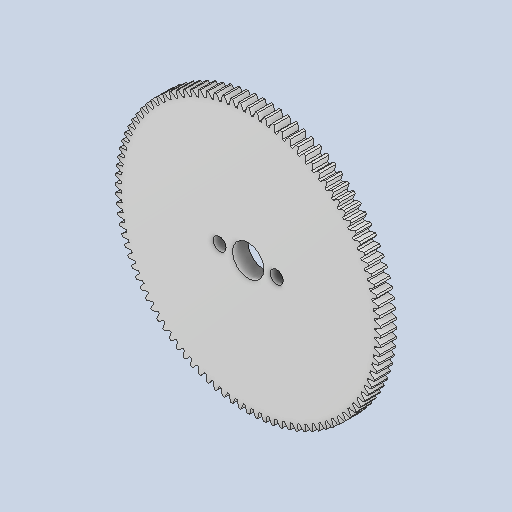
# Autodesk Inventor part: 平歯車1
Saved by Autodesk Inventor 2025.2 (Build 292293000, 293)
## iProperties
CustomPartVersion: 1
Created: 2025-01-13
Part Number: 平歯車1
Material: ABS プラスチック
Document SubType Name: Modeling
Designer: haruy
Categories: <?xml version="1.0" encoding="UTF-16"?> <MemberInstance><Categories><FamilyTemplate><FamilyTemplateParameter ValueType="xs:double" Id="1" ObjectReferenceKey="da_z" ObjectType="kUserParameterObject"/><FamilyTemplateParameter ValueType="xs:double" Id="2" ObjectReferenceKey="da_b" ObjectType="kUserParameterObject"/><FamilyTemplateParameter ValueType="xs:double" Id="3" ObjectReferenceKey="da_beta" ObjectType="kUserParameterObject"/><FamilyTemplateParameter ValueType="xs:double" Id="4" ObjectReferenceKey="da_da" ObjectType="kUserParameterObject"/><FamilyTemplateParameter ValueType="xs:double" Id="5" ObjectReferenceKey="da_aw" ObjectType="kUserParameterObject"/><FamilyTemplateParameter ValueType="xs:string" Id="6" ObjectReferenceKey="EAIAABAAAACIAQAAAAAAAIAAAAAAAAAA" ObjectType="83910656" SubObjectId="SurfaceGeometry"/></FamilyTemplate><ParamToTemplateMap><ParamToTemplate CategoryParameter="//CategoryParameter[@InternalName='046C89C9-8512-4d59-83FE-43B91F4F132A']" TemplateParameter="1"/><ParamToTemplate CategoryParameter="//CategoryParameter[@InternalName='2552DF32-E462-4b46-AEBF-C6C7768E72AC']" TemplateParameter="2"/><ParamToTemplate CategoryParameter="//CategoryParameter[@InternalName='C9EE641D-15FC-4fae-A226-E94C4372FDD7']" TemplateParameter="3"/><ParamToTemplate><ParamToTemplate CategoryParameter="//CategoryParameter[@InternalName='00B6519A-459B-49c7-AD84-2E56D39A5744']" ConstantValue="0.000000"/></ParamToTemplate><ParamToTemplate><ParamToTemplate CategoryParameter="//CategoryParameter[@InternalName='04B31F0E-C7A6-4894-AA32-9629BEFACF47']" ConstantValue="1.000000"/></ParamToTemplate><ParamToTemplate><ParamToTemplate CategoryParameter="//CategoryParameter[@InternalName='43CBEC2E-7847-49e7-A936-2F7889FCB2D9']" ConstantValue="0.250000"/></ParamToTemplate><ParamToTemplate><ParamToTemplate CategoryParameter="//CategoryParameter[@InternalName='B1EFC894-105D-4ebd-86BF-FA20ED196853']" ConstantValue="0.350000"/></ParamToTemplate><ParamToTemplate><ParamToTemplate CategoryParameter="//CategoryParameter[@InternalName='51175063-3D10-4879-93E8-6246FE8B403D']" ConstantValue="2060000000.000000"/></ParamToTemplate><ParamToTemplate><ParamToTemplate CategoryParameter="//CategoryParameter[@InternalName='A3A52E27-4454-46a9-B0BD-C932399B70AF']" ConstantValue="0.300000"/></ParamToTemplate><ParamToTemplate><ParamToTemplate CategoryParameter="//CategoryParameter[@InternalName='91B76062-C214-41d9-B1B9-14D2AB99603D']" ConstantValue="0.100000"/></ParamToTemplate><ParamToTemplate><ParamToTemplate CategoryParameter="//CategoryParameter[@InternalName='374E806E-8B8A-4dda-A9AA-1039D6500AD2']" ConstantValue="10.000000"/></ParamToTemplate><ParamToTemplate><ParamToTemplate CategoryParameter="//CategoryParameter[@InternalName='2D373A89-B862-43d6-8D0B-0CBF12AB9F6C']" ConstantValue="0.349066"/></ParamToTemplate><ParamToTemplate CategoryParameter="//CategoryParameter[@InternalName='37777632-D6A2-4fac-9D53-DB8ACD95C989']" TemplateParameter="4"/><ParamToTemplate CategoryParameter="//CategoryParameter[@InternalName='FD1017F1-B727-4f7e-9707-0F86F1FF9423']" TemplateParameter="5"/><ParamToTemplate><ParamToTemplate CategoryParameter="//CategoryParameter[@InternalName='9E1B4470-B2D3-4ff1-B813-535BB4CDF51A']" ConstantValue="3520000.000000"/></ParamToTemplate><ParamToTemplate><ParamToTemplate CategoryParameter="//CategoryParameter[@InternalName='F8452263-BFF6-458c-9FB1-07C4B99E95CD']" ConstantValue="11400000.000000"/></ParamToTemplate><ParamToTemplate><ParamToTemplate CategoryParameter="//CategoryParameter[@InternalName='3E3BB259-FD49-497f-8171-6EBC954A3479']" ConstantValue="2.000000"/></ParamToTemplate><ParamToTemplate CategoryParameter="//CategoryParameter[@InternalName='27C3BAF2-7550-4e4b-AE2C-0DB134B7D9B7']" TemplateParameter="6"/></ParamToTemplateMap><Category DisplayName="Gear" InternalName="DC85795E-93AB-48d5-8EEE-5A27447B64BD" Mnemonic="Gear"><CategoryParameter DisplayName="z" InternalName="046C89C9-8512-4d59-83FE-43B91F4F132A" Mnemonic="z"/><CategoryParameter DisplayName="b" InternalName="2552DF32-E462-4b46-AEBF-C6C7768E72AC" Mnemonic="b"/><CategoryParameter DisplayName="||b|" InternalName="C9EE641D-15FC-4fae-A226-E94C4372FDD7" Mnemonic="beta"/><CategoryParameter DisplayName="x" InternalName="00B6519A-459B-49c7-AD84-2E56D39A5744" Mnemonic="x"/><CategoryParameter DisplayName="a*" InternalName="04B31F0E-C7A6-4894-AA32-9629BEFACF47" Mnemonic="a"/><CategoryParameter DisplayName="c*" InternalName="43CBEC2E-7847-49e7-A936-2F7889FCB2D9" Mnemonic="c"/><CategoryParameter DisplayName="r|.f|*" InternalName="B1EFC894-105D-4ebd-86BF-FA20ED196853" Mnemonic="rf"/><CategoryParameter DisplayName="E" InternalName="51175063-3D10-4879-93E8-6246FE8B403D" Mnemonic="E"/><CategoryParameter DisplayName="||m|" InternalName="A3A52E27-4454-46a9-B0BD-C932399B70AF" Mnemonic="mi"/><Category DisplayName="SpurGear" InternalName="26C5A22E-A91E-4dfd-A3B3-23CCAFAE1764" Mnemonic="SpurGear"><CategoryParameter DisplayName="m" InternalName="91B76062-C214-41d9-B1B9-14D2AB99603D" Mnemonic="m"/><CategoryParameter DisplayName="P" InternalName="374E806E-8B8A-4dda-A9AA-1039D6500AD2" Mnemonic="PP"/><CategoryParameter DisplayName="||a|" InternalName="2D373A89-B862-43d6-8D0B-0CBF12AB9F6C" Mnemonic="alpha"/><CategoryParameter DisplayName="d|.a|" InternalName="37777632-D6A2-4fac-9D53-DB8ACD95C989" Mnemonic="da"/><CategoryParameter DisplayName="a|.w|" InternalName="FD1017F1-B727-4f7e-9707-0F86F1FF9423" Mnemonic="aw"/><CategoryParameter DisplayName="||s||.Flim|" InternalName="9E1B4470-B2D3-4ff1-B813-535BB4CDF51A" Mnemonic="sFlim"/><CategoryParameter DisplayName="||s||.Hlim|" InternalName="F8452263-BFF6-458c-9FB1-07C4B99E95CD" Mnemonic="sHlim"/><CategoryParameter DisplayName="タイプ" InternalName="3E3BB259-FD49-497f-8171-6EBC954A3479" Mnemonic="type"/><CategoryParameter DisplayName="PitchDiameter" InternalName="27C3BAF2-7550-4e4b-AE2C-0DB134B7D9B7" Mnemonic="IDS_PITCHDIAM"/></Category></Category></Categories></MemberInstance>
Density: 1.06 g/cm^3
Appearance: 滑らか - 白
Author: haruy
Autodesk Inventor part; units mm, degrees
ref_plane "YZ Plane" through (0, 0, 0) normal (1, 0, 0) x (0, 1, 0)
ref_plane "XZ Plane" through (0, 0, 0) normal (0, 1, 0) x (-1, 0, 0)
ref_plane "XY Plane" through (0, 0, 0) normal (0, 0, 1) x (1, 0, 0)
sketch "Sketch1" plane through (0, 0, 0) normal (0, 0, 1) x (1, 0, 0)
  circle A0 centre (0, 0) radius 51
  dimension "d0" = 102
  constraints: 1 centre point
  measures "d0" diameter of A0
extrude "Extrusion1" add sketch "Sketch1" along normal blind 6
ref_plane "Work Plane2" through (0, 0, 3) normal (0, 0, 1) x (1, 0, 0)
sketch "Sketch2" plane through (0, 0, 0) normal (0, 0, -1) x (-1, 0, 0)
  circle A0 centre (0, 0) radius 51 projected
  circle A1 centre (0, 0) radius 50
  dimension "d3" = 100
  constraints: 1 centre point, 1 coincident
  measures "d3" diameter of A1
surface extrude "ピッチ円直径" sketch "Sketch2" against normal through all shown no curves A1
ref_plane "Work Plane8" through (0, 0, 0) normal (0.9995066, 0.0314108, 0) x (0, 0, 1)
ref_plane "Work Plane9" through (0, 0, 0) normal (1, 0, 0) x (0, 1, 0)
spur gear teeth "平歯車" teeth 100 pitch diameter 100 tip diameter 102 root diameter 97.5 face width 6 start plane through (0, 0, 0) normal (0, 0, -1) x (-1, 0, 0)
sketch "スケッチ3" plane through (0, 0, 6) normal (0, 0, 1) x (1, 0, 0)
  circle A0 centre (0, 0) radius 6
  circle A1 centre (0, 0) radius 11
  circle A2 centre (-11, 0) radius 2.5
  circle A3 centre (11, 0) radius 2.5
  dimension "d50" = 22
  dimension "d49" = 12
  dimension "d51" = 5
  dimension "d54" = 360
  constraints: 3 centre point, 2 coincident, 1 horizontal alignment, 7 other
  measures "d49" diameter of A0
  measures "d51" diameter of A2
extrude "押し出し2" cut sketch "スケッチ3" against normal blind 10 contours A0 | A1 A3 | A1 A3 | A2 A1 | A1 A2
sketch "スケッチ4" plane through (0, 0, 6) normal (0, 0, 1) x (1, 0, 0)
  circle A0 centre (11, 0) radius 2.5 projected
  circle A1 centre (-11, 0) radius 2.5 projected
  circle A2 centre (0, 0) radius 6 projected
  arc A3 (-3.602, 50.8726) -> (-4.2065, 48.5682) centre (9.678, 46.1577) ccw projected
  arc A4 (-4.2065, 48.5682) -> (-4.9688, 48.4961) centre (0, 0) ccw projected
  arc A5 (-4.9688, 48.4961) -> (-5.9944, 50.6465) centre (-18.1557, 43.5266) ccw projected
  arc A6 (-5.9944, 50.6465) -> (-6.7892, 50.5461) centre (0, 0) ccw projected
  arc A7 (-6.7892, 50.5461) -> (-7.2478, 48.2082) centre (6.7606, 46.6743) ccw projected
  arc A8 (-7.2478, 48.2082) -> (-8.0041, 48.0884) centre (0, 0) ccw projected
  arc A9 (-8.0041, 48.0884) -> (-9.1627, 50.1702) centre (-20.8529, 42.3007) ccw projected
  arc A10 (-9.1627, 50.1702) -> (-9.9496, 50.02) centre (0, 0) ccw projected
  arc A11 (-9.9496, 50.02) -> (-10.2605, 47.658) centre (3.8166, 47.0067) ccw projected
  arc A12 (-10.2605, 47.658) -> (-11.0078, 47.491) centre (0, 0) ccw projected
  arc A13 (-11.0078, 47.491) -> (-12.2948, 49.4958) centre (-23.4678, 40.9079) ccw projected
  arc A14 (-12.2948, 49.4958) -> (-13.0708, 49.2966) centre (0, 0) ccw projected
  arc A15 (-13.0708, 49.2966) -> (-13.2327, 46.9197) centre (0.8575, 47.1536) ccw projected
  arc A16 (-13.2327, 46.9197) -> (-13.9681, 46.7061) centre (0, 0) ccw projected
  arc A17 (-13.9681, 46.7061) -> (-15.3784, 48.6262) centre (-25.9901, 39.3536) ccw projected
  arc A18 (-15.3784, 48.6262) -> (-16.1403, 48.3786) centre (0, 0) ccw projected
  arc A19 (-16.1403, 48.3786) -> (-16.1527, 45.9962) centre (-2.105, 47.1143) ccw projected
  arc A20 (-16.1527, 45.9962) -> (-16.8732, 45.7368) centre (0, 0) ccw projected
  arc A21 (-16.8732, 45.7368) -> (-18.4014, 47.5646) centre (-28.4099, 37.644) ccw projected
  arc A22 (-18.4014, 47.5646) -> (-19.1462, 47.2697) centre (0, 0) ccw projected
  arc A23 (-19.1462, 47.2697) -> (-19.009, 44.8912) centre (-5.0592, 46.8892) ccw projected
  arc A24 (-19.009, 44.8912) -> (-19.7118, 44.5871) centre (0, 0) ccw projected
  arc A25 (-19.7118, 44.5871) -> (-21.3516, 46.3153) centre (-30.7175, 35.7859) ccw projected
  arc A26 (-21.3516, 46.3153) -> (-22.0765, 45.9742) centre (0, 0) ccw projected
  arc A27 (-22.0765, 45.9742) -> (-21.7902, 43.6091) centre (-7.9934, 46.479) ccw projected
  arc A28 (-21.7902, 43.6091) -> (-22.4725, 43.2614) centre (0, 0) ccw projected
  arc A29 (-22.4725, 43.2614) -> (-24.2177, 44.8832) centre (-32.9039, 33.7865) ccw projected
  arc A30 (-24.2177, 44.8832) -> (-24.9197, 44.4973) centre (0, 0) ccw projected
  arc A31 (-24.9197, 44.4973) -> (-24.4854, 42.1548) centre (-10.8961, 45.8854) ccw projected
  arc A32 (-24.4854, 42.1548) -> (-25.1446, 41.765) centre (0, 0) ccw projected
  arc A33 (-25.1446, 41.765) -> (-26.9881, 43.274) centre (-34.9605, 31.6537) ccw projected
  arc A34 (-26.9881, 43.274) -> (-27.6645, 42.8448) centre (0, 0) ccw projected
  arc A35 (-27.6645, 42.8448) -> (-27.084, 40.5341) centre (-13.7557, 45.1107) ccw projected
  arc A36 (-27.084, 40.5341) -> (-27.7174, 40.1037) centre (0, 0) ccw projected
  arc A37 (-27.7174, 40.1037) -> (-29.6521, 41.494) centre (-36.879, 29.3961) ccw projected
  arc A38 (-29.6521, 41.494) -> (-30.3002, 41.0232) centre (0, 0) ccw projected
  arc A39 (-30.3002, 41.0232) -> (-29.5758, 38.7535) centre (-16.5611, 44.1579) ccw projected
  arc A40 (-29.5758, 38.7535) -> (-30.1808, 38.2842) centre (0, 0) ccw projected
  arc A41 (-30.1808, 38.2842) -> (-32.199, 39.5503) centre (-38.652, 27.0224) ccw projected
  arc A42 (-32.199, 39.5503) -> (-32.8162, 39.0396) centre (0, 0) ccw projected
  arc A43 (-32.8162, 39.0396) -> (-31.9508, 36.82) centre (-19.3011, 43.0309) ccw projected
  arc A44 (-31.9508, 36.82) -> (-32.5252, 36.3136) centre (0, 0) ccw projected
  arc A45 (-32.5252, 36.3136) -> (-34.6188, 37.4504) centre (-40.2725, 24.5421) ccw projected
  arc A46 (-34.6188, 37.4504) -> (-35.2028, 36.9021) centre (0, 0) ccw projected
  arc A47 (-35.2028, 36.9021) -> (-34.1997, 34.7411) centre (-21.965, 41.7341) ccw projected
  arc A48 (-34.1997, 34.7411) -> (-34.7411, 34.1997) centre (0, 0) ccw projected
  arc A49 (-34.7411, 34.1997) -> (-36.9021, 35.2028) centre (-41.7341, 21.965) ccw projected
  arc A50 (-36.9021, 35.2028) -> (-37.4504, 34.6188) centre (0, 0) ccw projected
  arc A51 (-37.4504, 34.6188) -> (-36.3136, 32.5252) centre (-24.5421, 40.2725) ccw projected
  arc A52 (-36.3136, 32.5252) -> (-36.82, 31.9508) centre (0, 0) ccw projected
  arc A53 (-36.82, 31.9508) -> (-39.0396, 32.8162) centre (-43.0309, 19.3011) ccw projected
  arc A54 (-39.0396, 32.8162) -> (-39.5503, 32.199) centre (0, 0) ccw projected
  arc A55 (-39.5503, 32.199) -> (-38.2842, 30.1808) centre (-27.0224, 38.652) ccw projected
  arc A56 (-38.2842, 30.1808) -> (-38.7535, 29.5758) centre (0, 0) ccw projected
  arc A57 (-38.7535, 29.5758) -> (-41.0232, 30.3002) centre (-44.1579, 16.5611) ccw projected
  arc A58 (-41.0232, 30.3002) -> (-41.494, 29.6521) centre (0, 0) ccw projected
  arc A59 (-41.494, 29.6521) -> (-40.1037, 27.7174) centre (-29.3961, 36.879) ccw projected
  arc A60 (-40.1037, 27.7174) -> (-40.5341, 27.084) centre (0, 0) ccw projected
  arc A61 (-40.5341, 27.084) -> (-42.8448, 27.6645) centre (-45.1107, 13.7557) ccw projected
  arc A62 (-42.8448, 27.6645) -> (-43.274, 26.9881) centre (0, 0) ccw projected
  arc A63 (-43.274, 26.9881) -> (-41.765, 25.1446) centre (-31.6537, 34.9605) ccw projected
  arc A64 (-41.765, 25.1446) -> (-42.1548, 24.4854) centre (0, 0) ccw projected
  arc A65 (-42.1548, 24.4854) -> (-44.4973, 24.9197) centre (-45.8854, 10.8961) ccw projected
  arc A66 (-44.4973, 24.9197) -> (-44.8832, 24.2177) centre (0, 0) ccw projected
  arc A67 (-44.8832, 24.2177) -> (-43.2614, 22.4725) centre (-33.7865, 32.9039) ccw projected
  arc A68 (-43.2614, 22.4725) -> (-43.6091, 21.7902) centre (0, 0) ccw projected
  arc A69 (-43.6091, 21.7902) -> (-45.9742, 22.0765) centre (-46.479, 7.9934) ccw projected
  arc A70 (-45.9742, 22.0765) -> (-46.3153, 21.3516) centre (0, 0) ccw projected
  arc A71 (-46.3153, 21.3516) -> (-44.5871, 19.7118) centre (-35.7859, 30.7175) ccw projected
  arc A72 (-44.5871, 19.7118) -> (-44.8912, 19.009) centre (0, 0) ccw projected
  arc A73 (-44.8912, 19.009) -> (-47.2697, 19.1462) centre (-46.8892, 5.0592) ccw projected
  arc A74 (-47.2697, 19.1462) -> (-47.5646, 18.4014) centre (0, 0) ccw projected
  arc A75 (-47.5646, 18.4014) -> (-45.7368, 16.8732) centre (-37.644, 28.4099) ccw projected
  arc A76 (-45.7368, 16.8732) -> (-45.9962, 16.1527) centre (0, 0) ccw projected
  arc A77 (-45.9962, 16.1527) -> (-48.3786, 16.1403) centre (-47.1143, 2.105) ccw projected
  arc A78 (-48.3786, 16.1403) -> (-48.6262, 15.3784) centre (0, 0) ccw projected
  arc A79 (-48.6262, 15.3784) -> (-46.7061, 13.9681) centre (-39.3536, 25.9901) ccw projected
  arc A80 (-46.7061, 13.9681) -> (-46.9197, 13.2327) centre (0, 0) ccw projected
  arc A81 (-46.9197, 13.2327) -> (-49.2966, 13.0708) centre (-47.1536, -0.8575) ccw projected
  arc A82 (-49.2966, 13.0708) -> (-49.4958, 12.2948) centre (0, 0) ccw projected
  arc A83 (-49.4958, 12.2948) -> (-47.491, 11.0078) centre (-40.9079, 23.4678) ccw projected
  arc A84 (-47.491, 11.0078) -> (-47.658, 10.2605) centre (0, 0) ccw projected
  arc A85 (-47.658, 10.2605) -> (-50.02, 9.9496) centre (-47.0067, -3.8166) ccw projected
  arc A86 (-50.02, 9.9496) -> (-50.1702, 9.1627) centre (0, 0) ccw projected
  arc A87 (-50.1702, 9.1627) -> (-48.0884, 8.0041) centre (-42.3007, 20.8529) ccw projected
  arc A88 (-48.0884, 8.0041) -> (-48.2082, 7.2478) centre (0, 0) ccw projected
  arc A89 (-48.2082, 7.2478) -> (-50.5461, 6.7892) centre (-46.6743, -6.7606) ccw projected
  arc A90 (-50.5461, 6.7892) -> (-50.6465, 5.9944) centre (0, 0) ccw projected
  arc A91 (-50.6465, 5.9944) -> (-48.4961, 4.9688) centre (-43.5266, 18.1557) ccw projected
  arc A92 (-48.4961, 4.9688) -> (-48.5682, 4.2065) centre (0, 0) ccw projected
  arc A93 (-48.5682, 4.2065) -> (-50.8726, 3.602) centre (-46.1577, -9.678) ccw projected
  arc A94 (-50.8726, 3.602) -> (-50.9229, 2.8025) centre (0, 0) ccw projected
  arc A95 (-50.9229, 2.8025) -> (-48.7124, 1.9139) centre (-44.5807, 15.3868) ccw projected
  arc A96 (-48.7124, 1.9139) -> (-48.7365, 1.1485) centre (0, 0) ccw projected
  arc A97 (-48.7365, 1.1485) -> (-50.9984, 0.4005) centre (-45.4589, -12.5572) ccw projected
  arc A98 (-50.9984, 0.4005) -> (-50.9984, -0.4005) centre (0, 0) ccw projected
  arc A99 (-50.9984, -0.4005) -> (-48.7365, -1.1485) centre (-45.4589, 12.5572) ccw projected
  arc A100 (-48.7365, -1.1485) -> (-48.7124, -1.9139) centre (0, 0) ccw projected
  arc A101 (-48.7124, -1.9139) -> (-50.9229, -2.8025) centre (-44.5807, -15.3868) ccw projected
  arc A102 (-50.9229, -2.8025) -> (-50.8726, -3.602) centre (0, 0) ccw projected
  arc A103 (-50.8726, -3.602) -> (-48.5682, -4.2065) centre (-46.1577, 9.678) ccw projected
  arc A104 (-48.5682, -4.2065) -> (-48.4961, -4.9688) centre (0, 0) ccw projected
  arc A105 (-48.4961, -4.9688) -> (-50.6465, -5.9944) centre (-43.5266, -18.1557) ccw projected
  arc A106 (-50.6465, -5.9944) -> (-50.5461, -6.7892) centre (0, 0) ccw projected
  arc A107 (-50.5461, -6.7892) -> (-48.2082, -7.2478) centre (-46.6743, 6.7606) ccw projected
  arc A108 (-48.2082, -7.2478) -> (-48.0884, -8.0041) centre (0, 0) ccw projected
  arc A109 (-48.0884, -8.0041) -> (-50.1702, -9.1627) centre (-42.3007, -20.8529) ccw projected
  arc A110 (-50.1702, -9.1627) -> (-50.02, -9.9496) centre (0, 0) ccw projected
  arc A111 (-50.02, -9.9496) -> (-47.658, -10.2605) centre (-47.0067, 3.8166) ccw projected
  arc A112 (-47.658, -10.2605) -> (-47.491, -11.0078) centre (0, 0) ccw projected
  arc A113 (-47.491, -11.0078) -> (-49.4958, -12.2948) centre (-40.9079, -23.4678) ccw projected
  arc A114 (-49.4958, -12.2948) -> (-49.2966, -13.0708) centre (0, 0) ccw projected
  arc A115 (-49.2966, -13.0708) -> (-46.9197, -13.2327) centre (-47.1536, 0.8575) ccw projected
  arc A116 (-46.9197, -13.2327) -> (-46.7061, -13.9681) centre (0, 0) ccw projected
  arc A117 (-46.7061, -13.9681) -> (-48.6262, -15.3784) centre (-39.3536, -25.9901) ccw projected
  arc A118 (-48.6262, -15.3784) -> (-48.3786, -16.1403) centre (0, 0) ccw projected
  arc A119 (-48.3786, -16.1403) -> (-45.9962, -16.1527) centre (-47.1143, -2.105) ccw projected
  arc A120 (-45.9962, -16.1527) -> (-45.7368, -16.8732) centre (0, 0) ccw projected
  arc A121 (-45.7368, -16.8732) -> (-47.5646, -18.4014) centre (-37.644, -28.4099) ccw projected
  arc A122 (-47.5646, -18.4014) -> (-47.2697, -19.1462) centre (0, 0) ccw projected
  arc A123 (-47.2697, -19.1462) -> (-44.8912, -19.009) centre (-46.8892, -5.0592) ccw projected
  arc A124 (-44.8912, -19.009) -> (-44.5871, -19.7118) centre (0, 0) ccw projected
  arc A125 (-44.5871, -19.7118) -> (-46.3153, -21.3516) centre (-35.7859, -30.7175) ccw projected
  arc A126 (-46.3153, -21.3516) -> (-45.9742, -22.0765) centre (0, 0) ccw projected
  arc A127 (-45.9742, -22.0765) -> (-43.6091, -21.7902) centre (-46.479, -7.9934) ccw projected
  arc A128 (-43.6091, -21.7902) -> (-43.2614, -22.4725) centre (0, 0) ccw projected
  arc A129 (-43.2614, -22.4725) -> (-44.8832, -24.2177) centre (-33.7865, -32.9039) ccw projected
  arc A130 (-44.8832, -24.2177) -> (-44.4973, -24.9197) centre (0, 0) ccw projected
  arc A131 (-44.4973, -24.9197) -> (-42.1548, -24.4854) centre (-45.8854, -10.8961) ccw projected
  arc A132 (-42.1548, -24.4854) -> (-41.765, -25.1446) centre (0, 0) ccw projected
  arc A133 (-41.765, -25.1446) -> (-43.274, -26.9881) centre (-31.6537, -34.9605) ccw projected
  arc A134 (-43.274, -26.9881) -> (-42.8448, -27.6645) centre (0, 0) ccw projected
  arc A135 (-42.8448, -27.6645) -> (-40.5341, -27.084) centre (-45.1107, -13.7557) ccw projected
  arc A136 (-40.5341, -27.084) -> (-40.1037, -27.7174) centre (0, 0) ccw projected
  arc A137 (-40.1037, -27.7174) -> (-41.494, -29.6521) centre (-29.3961, -36.879) ccw projected
  arc A138 (-41.494, -29.6521) -> (-41.0232, -30.3002) centre (0, 0) ccw projected
  arc A139 (-41.0232, -30.3002) -> (-38.7535, -29.5758) centre (-44.1579, -16.5611) ccw projected
  arc A140 (-38.7535, -29.5758) -> (-38.2842, -30.1808) centre (0, 0) ccw projected
  arc A141 (-38.2842, -30.1808) -> (-39.5503, -32.199) centre (-27.0224, -38.652) ccw projected
  arc A142 (-39.5503, -32.199) -> (-39.0396, -32.8162) centre (0, 0) ccw projected
  arc A143 (-39.0396, -32.8162) -> (-36.82, -31.9508) centre (-43.0309, -19.3011) ccw projected
  arc A144 (-36.82, -31.9508) -> (-36.3136, -32.5252) centre (0, 0) ccw projected
  arc A145 (-36.3136, -32.5252) -> (-37.4504, -34.6188) centre (-24.5421, -40.2725) ccw projected
  arc A146 (-37.4504, -34.6188) -> (-36.9021, -35.2028) centre (0, 0) ccw projected
  arc A147 (-36.9021, -35.2028) -> (-34.7411, -34.1997) centre (-41.7341, -21.965) ccw projected
  arc A148 (-34.7411, -34.1997) -> (-34.1997, -34.7411) centre (0, 0) ccw projected
  arc A149 (-34.1997, -34.7411) -> (-35.2028, -36.9021) centre (-21.965, -41.7341) ccw projected
  arc A150 (-35.2028, -36.9021) -> (-34.6188, -37.4504) centre (0, 0) ccw projected
  arc A151 (-34.6188, -37.4504) -> (-32.5252, -36.3136) centre (-40.2725, -24.5421) ccw projected
  arc A152 (-32.5252, -36.3136) -> (-31.9508, -36.82) centre (0, 0) ccw projected
  arc A153 (-31.9508, -36.82) -> (-32.8162, -39.0396) centre (-19.3011, -43.0309) ccw projected
  arc A154 (-32.8162, -39.0396) -> (-32.199, -39.5503) centre (0, 0) ccw projected
  arc A155 (-32.199, -39.5503) -> (-30.1808, -38.2842) centre (-38.652, -27.0224) ccw projected
  arc A156 (-30.1808, -38.2842) -> (-29.5758, -38.7535) centre (0, 0) ccw projected
  arc A157 (-29.5758, -38.7535) -> (-30.3002, -41.0232) centre (-16.5611, -44.1579) ccw projected
  arc A158 (-30.3002, -41.0232) -> (-29.6521, -41.494) centre (0, 0) ccw projected
  arc A159 (-29.6521, -41.494) -> (-27.7174, -40.1037) centre (-36.879, -29.3961) ccw projected
  arc A160 (-27.7174, -40.1037) -> (-27.084, -40.5341) centre (0, 0) ccw projected
  arc A161 (-27.084, -40.5341) -> (-27.6645, -42.8448) centre (-13.7557, -45.1107) ccw projected
  arc A162 (-27.6645, -42.8448) -> (-26.9881, -43.274) centre (0, 0) ccw projected
  arc A163 (-26.9881, -43.274) -> (-25.1446, -41.765) centre (-34.9605, -31.6537) ccw projected
  arc A164 (-25.1446, -41.765) -> (-24.4854, -42.1548) centre (0, 0) ccw projected
  arc A165 (-24.4854, -42.1548) -> (-24.9197, -44.4973) centre (-10.8961, -45.8854) ccw projected
  arc A166 (-24.9197, -44.4973) -> (-24.2177, -44.8832) centre (0, 0) ccw projected
  arc A167 (-24.2177, -44.8832) -> (-22.4725, -43.2614) centre (-32.9039, -33.7865) ccw projected
  arc A168 (-22.4725, -43.2614) -> (-21.7902, -43.6091) centre (0, 0) ccw projected
  arc A169 (-21.7902, -43.6091) -> (-22.0765, -45.9742) centre (-7.9934, -46.479) ccw projected
  arc A170 (-22.0765, -45.9742) -> (-21.3516, -46.3153) centre (0, 0) ccw projected
  arc A171 (-21.3516, -46.3153) -> (-19.7118, -44.5871) centre (-30.7175, -35.7859) ccw projected
  arc A172 (-19.7118, -44.5871) -> (-19.009, -44.8912) centre (0, 0) ccw projected
  arc A173 (-19.009, -44.8912) -> (-19.1462, -47.2697) centre (-5.0592, -46.8892) ccw projected
  arc A174 (-19.1462, -47.2697) -> (-18.4014, -47.5646) centre (0, 0) ccw projected
  arc A175 (-18.4014, -47.5646) -> (-16.8732, -45.7368) centre (-28.4099, -37.644) ccw projected
  arc A176 (-16.8732, -45.7368) -> (-16.1527, -45.9962) centre (0, 0) ccw projected
  arc A177 (-16.1527, -45.9962) -> (-16.1403, -48.3786) centre (-2.105, -47.1143) ccw projected
  arc A178 (-16.1403, -48.3786) -> (-15.3784, -48.6262) centre (0, 0) ccw projected
  arc A179 (-15.3784, -48.6262) -> (-13.9681, -46.7061) centre (-25.9901, -39.3536) ccw projected
  arc A180 (-13.9681, -46.7061) -> (-13.2327, -46.9197) centre (0, 0) ccw projected
  arc A181 (-13.2327, -46.9197) -> (-13.0708, -49.2966) centre (0.8575, -47.1536) ccw projected
  arc A182 (-13.0708, -49.2966) -> (-12.2948, -49.4958) centre (0, 0) ccw projected
  arc A183 (-12.2948, -49.4958) -> (-11.0078, -47.491) centre (-23.4678, -40.9079) ccw projected
  arc A184 (-11.0078, -47.491) -> (-10.2605, -47.658) centre (0, 0) ccw projected
  arc A185 (-10.2605, -47.658) -> (-9.9496, -50.02) centre (3.8166, -47.0067) ccw projected
  arc A186 (-9.9496, -50.02) -> (-9.1627, -50.1702) centre (0, 0) ccw projected
  arc A187 (-9.1627, -50.1702) -> (-8.0041, -48.0884) centre (-20.8529, -42.3007) ccw projected
  arc A188 (-8.0041, -48.0884) -> (-7.2478, -48.2082) centre (0, 0) ccw projected
  arc A189 (-7.2478, -48.2082) -> (-6.7892, -50.5461) centre (6.7606, -46.6743) ccw projected
  arc A190 (-6.7892, -50.5461) -> (-5.9944, -50.6465) centre (0, 0) ccw projected
  arc A191 (-5.9944, -50.6465) -> (-4.9688, -48.4961) centre (-18.1557, -43.5266) ccw projected
  arc A192 (-4.9688, -48.4961) -> (-4.2065, -48.5682) centre (0, 0) ccw projected
  arc A193 (-4.2065, -48.5682) -> (-3.602, -50.8726) centre (9.678, -46.1577) ccw projected
  arc A194 (-3.602, -50.8726) -> (-2.8025, -50.9229) centre (0, 0) ccw projected
  arc A195 (-2.8025, -50.9229) -> (-1.9139, -48.7124) centre (-15.3868, -44.5807) ccw projected
  arc A196 (-1.9139, -48.7124) -> (-1.1485, -48.7365) centre (0, 0) ccw projected
  arc A197 (-1.1485, -48.7365) -> (-0.4005, -50.9984) centre (12.5572, -45.4589) ccw projected
  arc A198 (-0.4005, -50.9984) -> (0.4005, -50.9984) centre (0, 0) ccw projected
  arc A199 (0.4005, -50.9984) -> (1.1485, -48.7365) centre (-12.5572, -45.4589) ccw projected
  arc A200 (1.1485, -48.7365) -> (1.9139, -48.7124) centre (0, 0) ccw projected
  arc A201 (1.9139, -48.7124) -> (2.8025, -50.9229) centre (15.3868, -44.5807) ccw projected
  arc A202 (2.8025, -50.9229) -> (3.602, -50.8726) centre (0, 0) ccw projected
  arc A203 (3.602, -50.8726) -> (4.2065, -48.5682) centre (-9.678, -46.1577) ccw projected
  arc A204 (4.2065, -48.5682) -> (4.9688, -48.4961) centre (0, 0) ccw projected
  arc A205 (4.9688, -48.4961) -> (5.9944, -50.6465) centre (18.1557, -43.5266) ccw projected
  arc A206 (5.9944, -50.6465) -> (6.7892, -50.5461) centre (0, 0) ccw projected
  arc A207 (6.7892, -50.5461) -> (7.2478, -48.2082) centre (-6.7606, -46.6743) ccw projected
  arc A208 (7.2478, -48.2082) -> (8.0041, -48.0884) centre (0, 0) ccw projected
  arc A209 (8.0041, -48.0884) -> (9.1627, -50.1702) centre (20.8529, -42.3007) ccw projected
  arc A210 (9.1627, -50.1702) -> (9.9496, -50.02) centre (0, 0) ccw projected
  arc A211 (9.9496, -50.02) -> (10.2605, -47.658) centre (-3.8166, -47.0067) ccw projected
  arc A212 (10.2605, -47.658) -> (11.0078, -47.491) centre (0, 0) ccw projected
  arc A213 (11.0078, -47.491) -> (12.2948, -49.4958) centre (23.4678, -40.9079) ccw projected
  arc A214 (12.2948, -49.4958) -> (13.0708, -49.2966) centre (0, 0) ccw projected
  arc A215 (13.0708, -49.2966) -> (13.2327, -46.9197) centre (-0.8575, -47.1536) ccw projected
  arc A216 (13.2327, -46.9197) -> (13.9681, -46.7061) centre (0, 0) ccw projected
  arc A217 (13.9681, -46.7061) -> (15.3784, -48.6262) centre (25.9901, -39.3536) ccw projected
  arc A218 (15.3784, -48.6262) -> (16.1403, -48.3786) centre (0, 0) ccw projected
  arc A219 (16.1403, -48.3786) -> (16.1527, -45.9962) centre (2.105, -47.1143) ccw projected
  arc A220 (16.1527, -45.9962) -> (16.8732, -45.7368) centre (0, 0) ccw projected
  arc A221 (16.8732, -45.7368) -> (18.4014, -47.5646) centre (28.4099, -37.644) ccw projected
  arc A222 (18.4014, -47.5646) -> (19.1462, -47.2697) centre (0, 0) ccw projected
  arc A223 (19.1462, -47.2697) -> (19.009, -44.8912) centre (5.0592, -46.8892) ccw projected
  arc A224 (19.009, -44.8912) -> (19.7118, -44.5871) centre (0, 0) ccw projected
  arc A225 (19.7118, -44.5871) -> (21.3516, -46.3153) centre (30.7175, -35.7859) ccw projected
  arc A226 (21.3516, -46.3153) -> (22.0765, -45.9742) centre (0, 0) ccw projected
  arc A227 (22.0765, -45.9742) -> (21.7902, -43.6091) centre (7.9934, -46.479) ccw projected
  arc A228 (21.7902, -43.6091) -> (22.4725, -43.2614) centre (0, 0) ccw projected
  arc A229 (22.4725, -43.2614) -> (24.2177, -44.8832) centre (32.9039, -33.7865) ccw projected
  arc A230 (24.2177, -44.8832) -> (24.9197, -44.4973) centre (0, 0) ccw projected
  arc A231 (24.9197, -44.4973) -> (24.4854, -42.1548) centre (10.8961, -45.8854) ccw projected
  arc A232 (24.4854, -42.1548) -> (25.1446, -41.765) centre (0, 0) ccw projected
  arc A233 (25.1446, -41.765) -> (26.9881, -43.274) centre (34.9605, -31.6537) ccw projected
  arc A234 (26.9881, -43.274) -> (27.6645, -42.8448) centre (0, 0) ccw projected
  arc A235 (27.6645, -42.8448) -> (27.084, -40.5341) centre (13.7557, -45.1107) ccw projected
  arc A236 (27.084, -40.5341) -> (27.7174, -40.1037) centre (0, 0) ccw projected
  arc A237 (27.7174, -40.1037) -> (29.6521, -41.494) centre (36.879, -29.3961) ccw projected
  arc A238 (29.6521, -41.494) -> (30.3002, -41.0232) centre (0, 0) ccw projected
  arc A239 (30.3002, -41.0232) -> (29.5758, -38.7535) centre (16.5611, -44.1579) ccw projected
  arc A240 (29.5758, -38.7535) -> (30.1808, -38.2842) centre (0, 0) ccw projected
  arc A241 (30.1808, -38.2842) -> (32.199, -39.5503) centre (38.652, -27.0224) ccw projected
  arc A242 (32.199, -39.5503) -> (32.8162, -39.0396) centre (0, 0) ccw projected
  arc A243 (32.8162, -39.0396) -> (31.9508, -36.82) centre (19.3011, -43.0309) ccw projected
  arc A244 (31.9508, -36.82) -> (32.5252, -36.3136) centre (0, 0) ccw projected
  arc A245 (32.5252, -36.3136) -> (34.6188, -37.4504) centre (40.2725, -24.5421) ccw projected
  arc A246 (34.6188, -37.4504) -> (35.2028, -36.9021) centre (0, 0) ccw projected
  arc A247 (35.2028, -36.9021) -> (34.1997, -34.7411) centre (21.965, -41.7341) ccw projected
  arc A248 (34.1997, -34.7411) -> (34.7411, -34.1997) centre (0, 0) ccw projected
  arc A249 (34.7411, -34.1997) -> (36.9021, -35.2028) centre (41.7341, -21.965) ccw projected
  arc A250 (36.9021, -35.2028) -> (37.4504, -34.6188) centre (0, 0) ccw projected
  arc A251 (37.4504, -34.6188) -> (36.3136, -32.5252) centre (24.5421, -40.2725) ccw projected
  arc A252 (36.3136, -32.5252) -> (36.82, -31.9508) centre (0, 0) ccw projected
  arc A253 (36.82, -31.9508) -> (39.0396, -32.8162) centre (43.0309, -19.3011) ccw projected
  arc A254 (39.0396, -32.8162) -> (39.5503, -32.199) centre (0, 0) ccw projected
  arc A255 (39.5503, -32.199) -> (38.2842, -30.1808) centre (27.0224, -38.652) ccw projected
  arc A256 (38.2842, -30.1808) -> (38.7535, -29.5758) centre (0, 0) ccw projected
  arc A257 (38.7535, -29.5758) -> (41.0232, -30.3002) centre (44.1579, -16.5611) ccw projected
  arc A258 (41.0232, -30.3002) -> (41.494, -29.6521) centre (0, 0) ccw projected
  arc A259 (41.494, -29.6521) -> (40.1037, -27.7174) centre (29.3961, -36.879) ccw projected
  arc A260 (40.1037, -27.7174) -> (40.5341, -27.084) centre (0, 0) ccw projected
  arc A261 (40.5341, -27.084) -> (42.8448, -27.6645) centre (45.1107, -13.7557) ccw projected
  arc A262 (42.8448, -27.6645) -> (43.274, -26.9881) centre (0, 0) ccw projected
  arc A263 (43.274, -26.9881) -> (41.765, -25.1446) centre (31.6537, -34.9605) ccw projected
  arc A264 (41.765, -25.1446) -> (42.1548, -24.4854) centre (0, 0) ccw projected
  arc A265 (42.1548, -24.4854) -> (44.4973, -24.9197) centre (45.8854, -10.8961) ccw projected
  arc A266 (44.4973, -24.9197) -> (44.8832, -24.2177) centre (0, 0) ccw projected
  arc A267 (44.8832, -24.2177) -> (43.2614, -22.4725) centre (33.7865, -32.9039) ccw projected
  arc A268 (43.2614, -22.4725) -> (43.6091, -21.7902) centre (0, 0) ccw projected
  arc A269 (43.6091, -21.7902) -> (45.9742, -22.0765) centre (46.479, -7.9934) ccw projected
  arc A270 (45.9742, -22.0765) -> (46.3153, -21.3516) centre (0, 0) ccw projected
  arc A271 (46.3153, -21.3516) -> (44.5871, -19.7118) centre (35.7859, -30.7175) ccw projected
  arc A272 (44.5871, -19.7118) -> (44.8912, -19.009) centre (0, 0) ccw projected
  arc A273 (44.8912, -19.009) -> (47.2697, -19.1462) centre (46.8892, -5.0592) ccw projected
  arc A274 (47.2697, -19.1462) -> (47.5646, -18.4014) centre (0, 0) ccw projected
  arc A275 (47.5646, -18.4014) -> (45.7368, -16.8732) centre (37.644, -28.4099) ccw projected
  arc A276 (45.7368, -16.8732) -> (45.9962, -16.1527) centre (0, 0) ccw projected
  arc A277 (45.9962, -16.1527) -> (48.3786, -16.1403) centre (47.1143, -2.105) ccw projected
  arc A278 (48.3786, -16.1403) -> (48.6262, -15.3784) centre (0, 0) ccw projected
  arc A279 (48.6262, -15.3784) -> (46.7061, -13.9681) centre (39.3536, -25.9901) ccw projected
  arc A280 (46.7061, -13.9681) -> (46.9197, -13.2327) centre (0, 0) ccw projected
  arc A281 (46.9197, -13.2327) -> (49.2966, -13.0708) centre (47.1536, 0.8575) ccw projected
  arc A282 (49.2966, -13.0708) -> (49.4958, -12.2948) centre (0, 0) ccw projected
  arc A283 (49.4958, -12.2948) -> (47.491, -11.0078) centre (40.9079, -23.4678) ccw projected
  arc A284 (47.491, -11.0078) -> (47.658, -10.2605) centre (0, 0) ccw projected
  arc A285 (47.658, -10.2605) -> (50.02, -9.9496) centre (47.0067, 3.8166) ccw projected
  arc A286 (50.02, -9.9496) -> (50.1702, -9.1627) centre (0, 0) ccw projected
  arc A287 (50.1702, -9.1627) -> (48.0884, -8.0041) centre (42.3007, -20.8529) ccw projected
  arc A288 (48.0884, -8.0041) -> (48.2082, -7.2478) centre (0, 0) ccw projected
  arc A289 (48.2082, -7.2478) -> (50.5461, -6.7892) centre (46.6743, 6.7606) ccw projected
  arc A290 (50.5461, -6.7892) -> (50.6465, -5.9944) centre (0, 0) ccw projected
  arc A291 (50.6465, -5.9944) -> (48.4961, -4.9688) centre (43.5266, -18.1557) ccw projected
  arc A292 (48.4961, -4.9688) -> (48.5682, -4.2065) centre (0, 0) ccw projected
  arc A293 (48.5682, -4.2065) -> (50.8726, -3.602) centre (46.1577, 9.678) ccw projected
  arc A294 (50.8726, -3.602) -> (50.9229, -2.8025) centre (0, 0) ccw projected
  arc A295 (50.9229, -2.8025) -> (48.7124, -1.9139) centre (44.5807, -15.3868) ccw projected
  arc A296 (48.7124, -1.9139) -> (48.7365, -1.1485) centre (0, 0) ccw projected
  arc A297 (48.7365, -1.1485) -> (50.9984, -0.4005) centre (45.4589, 12.5572) ccw projected
  arc A298 (50.9984, -0.4005) -> (50.9984, 0.4005) centre (0, 0) ccw projected
  arc A299 (50.9984, 0.4005) -> (48.7365, 1.1485) centre (45.4589, -12.5572) ccw projected
  arc A300 (48.7365, 1.1485) -> (48.7124, 1.9139) centre (0, 0) ccw projected
  arc A301 (48.7124, 1.9139) -> (50.9229, 2.8025) centre (44.5807, 15.3868) ccw projected
  arc A302 (50.9229, 2.8025) -> (50.8726, 3.602) centre (0, 0) ccw projected
  arc A303 (50.8726, 3.602) -> (48.5682, 4.2065) centre (46.1577, -9.678) ccw projected
  arc A304 (48.5682, 4.2065) -> (48.4961, 4.9688) centre (0, 0) ccw projected
  arc A305 (48.4961, 4.9688) -> (50.6465, 5.9944) centre (43.5266, 18.1557) ccw projected
  arc A306 (50.6465, 5.9944) -> (50.5461, 6.7892) centre (0, 0) ccw projected
  arc A307 (50.5461, 6.7892) -> (48.2082, 7.2478) centre (46.6743, -6.7606) ccw projected
  arc A308 (48.2082, 7.2478) -> (48.0884, 8.0041) centre (0, 0) ccw projected
  arc A309 (48.0884, 8.0041) -> (50.1702, 9.1627) centre (42.3007, 20.8529) ccw projected
  arc A310 (50.1702, 9.1627) -> (50.02, 9.9496) centre (0, 0) ccw projected
  arc A311 (50.02, 9.9496) -> (47.658, 10.2605) centre (47.0067, -3.8166) ccw projected
  arc A312 (47.658, 10.2605) -> (47.491, 11.0078) centre (0, 0) ccw projected
  arc A313 (47.491, 11.0078) -> (49.4958, 12.2948) centre (40.9079, 23.4678) ccw projected
  arc A314 (49.4958, 12.2948) -> (49.2966, 13.0708) centre (0, 0) ccw projected
  arc A315 (49.2966, 13.0708) -> (46.9197, 13.2327) centre (47.1536, -0.8575) ccw projected
  arc A316 (46.9197, 13.2327) -> (46.7061, 13.9681) centre (0, 0) ccw projected
  arc A317 (46.7061, 13.9681) -> (48.6262, 15.3784) centre (39.3536, 25.9901) ccw projected
  arc A318 (48.6262, 15.3784) -> (48.3786, 16.1403) centre (0, 0) ccw projected
  arc A319 (48.3786, 16.1403) -> (45.9962, 16.1527) centre (47.1143, 2.105) ccw projected
  arc A320 (45.9962, 16.1527) -> (45.7368, 16.8732) centre (0, 0) ccw projected
  arc A321 (45.7368, 16.8732) -> (47.5646, 18.4014) centre (37.644, 28.4099) ccw projected
  arc A322 (47.5646, 18.4014) -> (47.2697, 19.1462) centre (0, 0) ccw projected
  arc A323 (47.2697, 19.1462) -> (44.8912, 19.009) centre (46.8892, 5.0592) ccw projected
  arc A324 (44.8912, 19.009) -> (44.5871, 19.7118) centre (0, 0) ccw projected
  arc A325 (44.5871, 19.7118) -> (46.3153, 21.3516) centre (35.7859, 30.7175) ccw projected
  arc A326 (46.3153, 21.3516) -> (45.9742, 22.0765) centre (0, 0) ccw projected
  arc A327 (45.9742, 22.0765) -> (43.6091, 21.7902) centre (46.479, 7.9934) ccw projected
  arc A328 (43.6091, 21.7902) -> (43.2614, 22.4725) centre (0, 0) ccw projected
  arc A329 (43.2614, 22.4725) -> (44.8832, 24.2177) centre (33.7865, 32.9039) ccw projected
  arc A330 (44.8832, 24.2177) -> (44.4973, 24.9197) centre (0, 0) ccw projected
  arc A331 (44.4973, 24.9197) -> (42.1548, 24.4854) centre (45.8854, 10.8961) ccw projected
  arc A332 (42.1548, 24.4854) -> (41.765, 25.1446) centre (0, 0) ccw projected
  arc A333 (41.765, 25.1446) -> (43.274, 26.9881) centre (31.6537, 34.9605) ccw projected
  arc A334 (43.274, 26.9881) -> (42.8448, 27.6645) centre (0, 0) ccw projected
  arc A335 (42.8448, 27.6645) -> (40.5341, 27.084) centre (45.1107, 13.7557) ccw projected
  arc A336 (40.5341, 27.084) -> (40.1037, 27.7174) centre (0, 0) ccw projected
  arc A337 (40.1037, 27.7174) -> (41.494, 29.6521) centre (29.3961, 36.879) ccw projected
  arc A338 (41.494, 29.6521) -> (41.0232, 30.3002) centre (0, 0) ccw projected
  arc A339 (41.0232, 30.3002) -> (38.7535, 29.5758) centre (44.1579, 16.5611) ccw projected
  arc A340 (38.7535, 29.5758) -> (38.2842, 30.1808) centre (0, 0) ccw projected
  arc A341 (38.2842, 30.1808) -> (39.5503, 32.199) centre (27.0224, 38.652) ccw projected
  arc A342 (39.5503, 32.199) -> (39.0396, 32.8162) centre (0, 0) ccw projected
  arc A343 (39.0396, 32.8162) -> (36.82, 31.9508) centre (43.0309, 19.3011) ccw projected
  arc A344 (36.82, 31.9508) -> (36.3136, 32.5252) centre (0, 0) ccw projected
  arc A345 (36.3136, 32.5252) -> (37.4504, 34.6188) centre (24.5421, 40.2725) ccw projected
  arc A346 (37.4504, 34.6188) -> (36.9021, 35.2028) centre (0, 0) ccw projected
  arc A347 (36.9021, 35.2028) -> (34.7411, 34.1997) centre (41.7341, 21.965) ccw projected
  arc A348 (34.7411, 34.1997) -> (34.1997, 34.7411) centre (0, 0) ccw projected
  arc A349 (34.1997, 34.7411) -> (35.2028, 36.9021) centre (21.965, 41.7341) ccw projected
  arc A350 (35.2028, 36.9021) -> (34.6188, 37.4504) centre (0, 0) ccw projected
  arc A351 (34.6188, 37.4504) -> (32.5252, 36.3136) centre (40.2725, 24.5421) ccw projected
  arc A352 (32.5252, 36.3136) -> (31.9508, 36.82) centre (0, 0) ccw projected
  arc A353 (31.9508, 36.82) -> (32.8162, 39.0396) centre (19.3011, 43.0309) ccw projected
  arc A354 (32.8162, 39.0396) -> (32.199, 39.5503) centre (0, 0) ccw projected
  arc A355 (32.199, 39.5503) -> (30.1808, 38.2842) centre (38.652, 27.0224) ccw projected
  arc A356 (30.1808, 38.2842) -> (29.5758, 38.7535) centre (0, 0) ccw projected
  arc A357 (29.5758, 38.7535) -> (30.3002, 41.0232) centre (16.5611, 44.1579) ccw projected
  arc A358 (30.3002, 41.0232) -> (29.6521, 41.494) centre (0, 0) ccw projected
  arc A359 (29.6521, 41.494) -> (27.7174, 40.1037) centre (36.879, 29.3961) ccw projected
  arc A360 (27.7174, 40.1037) -> (27.084, 40.5341) centre (0, 0) ccw projected
  arc A361 (27.084, 40.5341) -> (27.6645, 42.8448) centre (13.7557, 45.1107) ccw projected
  arc A362 (27.6645, 42.8448) -> (26.9881, 43.274) centre (0, 0) ccw projected
  arc A363 (26.9881, 43.274) -> (25.1446, 41.765) centre (34.9605, 31.6537) ccw projected
  arc A364 (25.1446, 41.765) -> (24.4854, 42.1548) centre (0, 0) ccw projected
  arc A365 (24.4854, 42.1548) -> (24.9197, 44.4973) centre (10.8961, 45.8854) ccw projected
  arc A366 (24.9197, 44.4973) -> (24.2177, 44.8832) centre (0, 0) ccw projected
  arc A367 (24.2177, 44.8832) -> (22.4725, 43.2614) centre (32.9039, 33.7865) ccw projected
  arc A368 (22.4725, 43.2614) -> (21.7902, 43.6091) centre (0, 0) ccw projected
  arc A369 (21.7902, 43.6091) -> (22.0765, 45.9742) centre (7.9934, 46.479) ccw projected
  arc A370 (22.0765, 45.9742) -> (21.3516, 46.3153) centre (0, 0) ccw projected
  arc A371 (21.3516, 46.3153) -> (19.7118, 44.5871) centre (30.7175, 35.7859) ccw projected
  arc A372 (19.7118, 44.5871) -> (19.009, 44.8912) centre (0, 0) ccw projected
  arc A373 (19.009, 44.8912) -> (19.1462, 47.2697) centre (5.0592, 46.8892) ccw projected
  arc A374 (19.1462, 47.2697) -> (18.4014, 47.5646) centre (0, 0) ccw projected
  arc A375 (18.4014, 47.5646) -> (16.8732, 45.7368) centre (28.4099, 37.644) ccw projected
  arc A376 (16.8732, 45.7368) -> (16.1527, 45.9962) centre (0, 0) ccw projected
  arc A377 (16.1527, 45.9962) -> (16.1403, 48.3786) centre (2.105, 47.1143) ccw projected
  arc A378 (16.1403, 48.3786) -> (15.3784, 48.6262) centre (0, 0) ccw projected
  arc A379 (15.3784, 48.6262) -> (13.9681, 46.7061) centre (25.9901, 39.3536) ccw projected
  arc A380 (13.9681, 46.7061) -> (13.2327, 46.9197) centre (0, 0) ccw projected
  arc A381 (13.2327, 46.9197) -> (13.0708, 49.2966) centre (-0.8575, 47.1536) ccw projected
  arc A382 (13.0708, 49.2966) -> (12.2948, 49.4958) centre (0, 0) ccw projected
  arc A383 (12.2948, 49.4958) -> (11.0078, 47.491) centre (23.4678, 40.9079) ccw projected
  arc A384 (11.0078, 47.491) -> (10.2605, 47.658) centre (0, 0) ccw projected
  arc A385 (10.2605, 47.658) -> (9.9496, 50.02) centre (-3.8166, 47.0067) ccw projected
  arc A386 (9.9496, 50.02) -> (9.1627, 50.1702) centre (0, 0) ccw projected
  arc A387 (9.1627, 50.1702) -> (8.0041, 48.0884) centre (20.8529, 42.3007) ccw projected
  arc A388 (8.0041, 48.0884) -> (7.2478, 48.2082) centre (0, 0) ccw projected
  arc A389 (7.2478, 48.2082) -> (6.7892, 50.5461) centre (-6.7606, 46.6743) ccw projected
  arc A390 (6.7892, 50.5461) -> (5.9944, 50.6465) centre (0, 0) ccw projected
  arc A391 (5.9944, 50.6465) -> (4.9688, 48.4961) centre (18.1557, 43.5266) ccw projected
  arc A392 (4.9688, 48.4961) -> (4.2065, 48.5682) centre (0, 0) ccw projected
  arc A393 (4.2065, 48.5682) -> (3.602, 50.8726) centre (-9.678, 46.1577) ccw projected
  arc A394 (3.602, 50.8726) -> (2.8025, 50.9229) centre (0, 0) ccw projected
  arc A395 (2.8025, 50.9229) -> (1.9139, 48.7124) centre (15.3868, 44.5807) ccw projected
  arc A396 (1.9139, 48.7124) -> (1.1485, 48.7365) centre (0, 0) ccw projected
  arc A397 (1.1485, 48.7365) -> (0.4005, 50.9984) centre (-12.5572, 45.4589) ccw projected
  arc A398 (0.4005, 50.9984) -> (-0.4005, 50.9984) centre (0, 0) ccw projected
  arc A399 (-0.4005, 50.9984) -> (-1.1485, 48.7365) centre (12.5572, 45.4589) ccw projected
  arc A400 (-1.1485, 48.7365) -> (-1.9139, 48.7124) centre (0, 0) ccw projected
  arc A401 (-1.9139, 48.7124) -> (-2.8025, 50.9229) centre (-15.3868, 44.5807) ccw projected
  arc A402 (-2.8025, 50.9229) -> (-3.602, 50.8726) centre (0, 0) ccw projected
equation "\"d0\" = da_da"
equation "\"d1\" = da_b"
equation "\"d3\" = da_d"
equation "\"d16\" = da_aw"
equation "\"d43\" = da_aw"
equation "\"d46\" = da_aw"
equation "\"da_da\" = 102"
equation "\"da_b\" = 6"
equation "\"da_d\" = 100"
equation "\"da_aw\" = 62.5"
body "Solid1"
body "Srf1"
